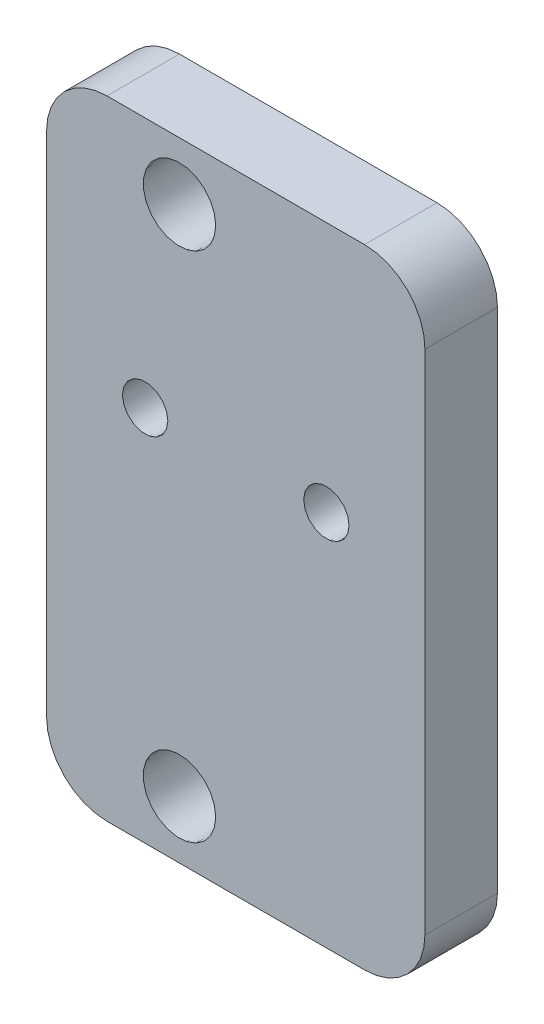
# Autodesk Inventor part: Switch on T nut holder
Saved by Autodesk Inventor 2018 (Build 220112000, 112)
## iProperties
Created: 2018-11-29
Part Number: Switch on T nut holder
Material: Generic
Document SubType Name: Modeling
Designer: ball
Density: 1 g/cm^3
Appearance: Default
Author: ball
Autodesk Inventor part; units mm, degrees
ref_plane "YZ Plane" through (0, 0, 0) normal (1, 0, 0) x (0, 1, 0)
ref_plane "XZ Plane" through (0, 0, 0) normal (0, 1, 0) x (-1, 0, 0)
ref_plane "XY Plane" through (0, 0, 0) normal (0, 0, 1) x (1, 0, 0)
ref_plane "Work Plane3" through (0, 0, 0) normal (0, 0, 1) x (1, 0, 0)
sketch "Sketch1" plane through (0, 0, 0) normal (0, 0, 1) x (1, 0, 0)
  line L0 (12.9032, 330.789) -> (12.9032, 321.137) projected
  line L1 (-6.985, 321.137) -> (-6.985, 330.0524) projected
  line L2 (3.1132, 307.8274) -> (-3.1132, 307.8274) projected
  line L3 (3.1132, 340.8474) -> (-3.1132, 340.8474) projected
  line L4 (12.9032, 340.8474) -> (-6.985, 340.8474)
  line L5 (-6.985, 340.8474) -> (-6.985, 307.8274)
  line L6 (-6.985, 307.8274) -> (12.9032, 307.8274)
  line L7 (12.9032, 307.8274) -> (12.9032, 340.8474)
  arc A0 (-1.7468, 337.6651) -> (-1.3298, 338.9494) centre (0, 337.8078) ccw
  arc A1 (-1.7468, 310.7243) -> (-1.3298, 312.0086) centre (0, 310.867) ccw
  circle A2 centre (0, 337.8078) radius 1.778
  point P0 (0, 0)
  dimension "d2" = 3.556
  constraints: 8 end point, 4 point on circle, 3 centre point, 2 parallel, 1 coincident, 1 horizontal, 1 perpendicular, 1 point on line, 8 other
  measures "d2" diameter of A2
ref_plane "Work Plane2" through (-6.985, 321.137, 5.08) normal (0, 0, -1) x (0, 1, 0)
extrude "Extrusion1" add sketch "Sketch1" along normal blind 3.81 contours L0 L7 L6 L2 L5 L1 L4 L3 | A2
sketch "Sketch3" plane through (-6.985, 340.8474, 3.81) normal (0, 0, 1) x (1, 0, 0)
  circle A0 centre (5.1816, -13.1996) radius 1.1938
  circle A1 centre (14.7066, -13.1996) radius 1.1938
  circle A2 centre (5.1816, -13.1996) radius 1.1938
  circle A3 centre (14.7066, -13.1996) radius 1.1938
  arc A4 (8.2018, -4.301) -> (6.9677, -4.7921) centre (6.985, -3.0396) ccw projected
  arc A5 (8.2018, -31.2417) -> (6.9677, -31.7329) centre (6.985, -29.9804) ccw projected
  circle A6 centre (6.985, -3.0396) radius 1.778
  circle A7 centre (6.985, -29.9804) radius 1.778
  arc A8 (8.2018, -31.2417) -> (6.9677, -31.7329) centre (6.985, -29.9804) ccw
  circle A9 centre (6.985, -29.9804) radius 1.778
  point P0 (6.985, -340.8474)
  dimension "d17" = 3.556
  dimension "d18" = 3.556
  dimension "d26" = 3.556
  dimension "d42" = 7.7216
  dimension "d43" = 1.8034
  dimension "d57" = 10.16
  dimension "d58" = 10.16
  constraints: 8 centre point, 5 coincident, 2 concentric, 2 point on circle, 4 other
  measures "d17" diameter of A6
  measures "d18" diameter of A7
  measures "d26" diameter of A9
  measures "d42" horizontal distance of A1.centre A5.centre
  measures "d43" horizontal distance of A0.centre A5.centre
  measures "d57" vertical distance of A1.centre A4.centre
  measures "d58" vertical distance of A4.centre A0.centre
sketch "Sketch4" plane through (0, 0, 0) normal (0, 0, -1) x (-1, 0, 0)
  circle A0 centre (1.8034, 323.5691) radius 1.1938 projected
  circle A1 centre (-7.7216, 323.5691) radius 1.1938 projected
  circle A2 centre (1.8034, 323.5691) radius 1.1938
  circle A3 centre (-7.7216, 323.5691) radius 1.1938
  point P0 (0, 0)
  constraints: 2 centre point, 2 coincident, 2 concentric
sketch "Sketch5" plane through (0, 0, 0) normal (0, 0, -1) x (-1, 0, 0)
  circle A0 centre (-7.7216, 323.5691) radius 1.1938 projected
  circle A1 centre (-7.7216, 323.5691) radius 1.1938 projected
  circle A2 centre (-7.7216, 323.5691) radius 1.1938
  point P0 (0, 0)
  constraints: 1 centre point, 1 coincident, 1 concentric
hole "Hole3" at (0, 337.8078, 3.81) direction (0, 0, -1) diameter 3.81 end through all
sketch "Sketch6" plane through (0, 0, 0) normal (0, 0, -1) x (-1, 0, 0)
  arc A0 (0.0173, 309.1145) -> (-1.2168, 309.6057) centre (0, 310.867) ccw projected
  circle A1 centre (0, 310.867) radius 1.778
  point P0 (0, 0)
  dimension "d27" = 3.556
  constraints: 1 centre point, 1 coincident
  measures "d27" diameter of A1
hole "Hole4" at (0, 310.867, 0) direction (0, 0, 1) diameter 3.81 end through all
fillet "Fillet5" radius 3.175 4 edges at (12.9032, 307.8274, 1.905) (-6.985, 307.8274, 1.905) (-6.985, 340.8474, 1.905) (12.9032, 340.8474, 1.905)
sketch "Sketch8" plane through (0, 0, 0) normal (0, 0, -1) x (-1, 0, 0)
  circle A0 centre (1.8034, 327.6478) radius 1.1938
  circle A1 centre (-7.7216, 327.6478) radius 1.1938
  circle A2 centre (0, 310.867) radius 1.905 projected
  circle A3 centre (0, 337.8078) radius 1.905 projected
  point P0 (0, 0)
  dimension "d44" = 2.3876
  dimension "d45" = 2.3876
  dimension "d47" = 1.8034
  dimension "d48" = 7.7216
  dimension "d59" = 10.16
  dimension "d60" = 10.16
  constraints: 2 centre point
  measures "d44" diameter of A0
  measures "d45" diameter of A1
  measures "d47" horizontal distance of A0.centre A2.centre
  measures "d48" horizontal distance of A1.centre A2.centre
  measures "d59" vertical distance of A3.centre A1.centre
  measures "d60" vertical distance of A3.centre A0.centre
hole "Hole5" at (-1.8034, 327.6478, 0) at (7.7216, 327.6478, 0) direction (0, 0, 1) diameter 2.3876 end through all counterbore diameter 5.08 counterbore depth 1.905
body "Solid1"
